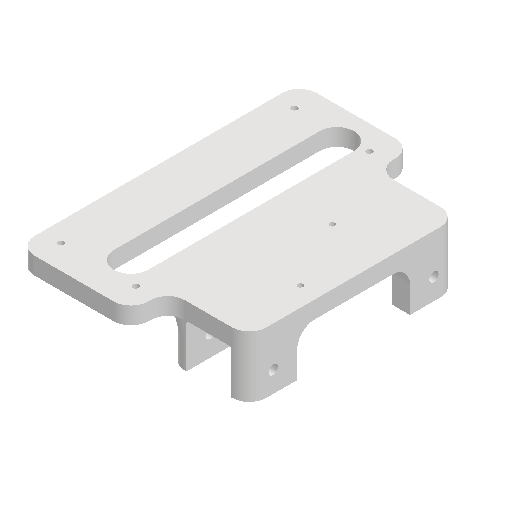
# Autodesk Inventor part: odriveAndBatteryMountV1
Saved by Autodesk Inventor 2025 (Build 290162000, 162)
## iProperties
Created: 2024-11-21
Part Number: odriveAndBatteryMountV1
Material: Generic
Document SubType Name: Modeling
Designer: derm
Density: 1 g/cm^3
Appearance: Default
Author: derm
Autodesk Inventor part; units mm, degrees
ref_plane "YZ Plane" through (0, 0, 0) normal (1, 0, 0) x (0, 1, 0)
ref_plane "XZ Plane" through (0, 0, 0) normal (0, 1, 0) x (-1, 0, 0)
ref_plane "XY Plane" through (0, 0, 0) normal (0, 0, 1) x (1, 0, 0)
sketch "Sketch1" plane through (0, 0, 0) normal (0, 1, 0) x (-1, 0, 0)
  line L0 (-21.75, 67.75) -> (21.75, 67.75) construction
  line L1 (21.75, 67.75) -> (21.75, -67.75) construction
  line L2 (21.75, -67.75) -> (-21.75, -67.75) construction
  line L3 (-21.75, -67.75) -> (-21.75, 67.75) construction
  line L4 (-21.75, 67.75) -> (21.75, -67.75) construction
  line L5 (21.75, 67.75) -> (-21.75, -67.75) construction
  line L6 (-32.9476, 81.798) -> (32.9476, 81.798)
  line L7 (32.9476, 81.798) -> (32.9476, -81.798)
  line L8 (32.9476, -81.798) -> (-32.9476, -81.798)
  line L9 (-32.9476, -81.798) -> (-32.9476, 81.798)
  line L10 (-32.9476, 81.798) -> (32.9476, -81.798) construction
  line L11 (32.9476, 81.798) -> (-32.9476, -81.798) construction
  circle A0 centre (21.75, 67.75) radius 1.75
  circle A1 centre (21.75, -67.75) radius 1.75
  circle A2 centre (-21.75, -67.75) radius 1.75
  circle A3 centre (-21.75, 67.75) radius 1.75
  line L12 (-31.798, -14.291) -> (-32.9476, -81.798)
  line L13 (-80.267, 60.5024) -> (-32.585, 60.5024)
  line L14 (-32.585, 60.5024) -> (-32.585, -60.5024)
  line L15 (-32.585, -60.5024) -> (-80.267, -60.5024)
  line L16 (-80.267, -60.5024) -> (-80.267, 60.5024)
  line L17 (-80.267, 60.5024) -> (-32.585, -60.5024) construction
  line L18 (-32.585, 60.5024) -> (-80.267, -60.5024) construction
  line L19 (-7.0609, 55.9115) -> (-7.0609, -63.5484) construction
  line L20 (-17.0051, 55.9115) -> (-17.0051, -63.5484)
  line L21 (2.8834, -63.5484) -> (2.8834, 55.9115)
  arc A4 (2.8834, 55.9115) -> (-17.0051, 55.9115) centre (-7.0609, 55.9115) ccw
  arc A5 (-17.0051, -63.5484) -> (2.8834, -63.5484) centre (-7.0609, -63.5484) ccw
  line L22 (32.9476, 81.798) -> (84.947, 81.798)
  line L23 (84.947, 81.798) -> (84.947, -81.798)
  line L24 (84.947, -81.798) -> (32.9476, -81.798)
  line L25 (32.9476, -81.798) -> (32.9476, 81.798)
  point P0 (0, 0)
  point P1 (-83.552, -67.75)
  point P2 (-56.426, 0)
  point P3 (-32.9476, -60.5024)
  point P4 (-32.9476, 60.5024)
  point P5 (-7.0609, -3.8185)
  dimension "d0" = 3.5
  dimension "d3" = 135.5
  dimension "d4" = 43.5
  constraints: 54 end point, 9 parallel, 7 midpoint, 6 centre point, 4 coincident, 4 horizontal, 4 perpendicular, 4 point on circle, 4 tangent, 3 equal radius, 2 point on line, 1 vertical, 1 other
  measures "d0" diameter of A3
  measures "d3" distance of L2.end L0.start
  measures "d4" distance of L0.start L0.end
extrude "Extrusion1" add sketch "Sketch1" against normal blind 10 contours L6 L7 L8 L12 L14 L13 L9 | L13 L14 L15 L9 | L9 L15 L16 L13
sketch "Sketch2" plane through (0, 0, 0) normal (0, 1, 0) x (1, 0, 0)
  circle A0 centre (69.0156, -19.6674) radius 1.6 projected
  circle A1 centre (47.6156, 20.3326) radius 1.6 projected
  point P0 (0, 0)
extrude "Extrusion2" cut sketch "Sketch2" against normal through all
sketch "Sketch3" plane through (0, -10, 0) normal (0, -1, 0) x (1, 0, 0)
  circle A0 centre (47.6156, -20.3326) radius 1.6 projected
  circle A1 centre (69.0156, 19.6674) radius 1.6 projected
  line L0 (32.585, -60.5024) -> (80.267, -60.5024) projected
  line L1 (80.267, -60.5024) -> (80.267, 60.5024) projected
  line L2 (80.267, 60.5024) -> (32.9476, 60.5024) projected
  line L3 (32.9476, 60.5024) -> (32.9476, 81.798) projected
  line L4 (32.9476, 81.798) -> (-32.9476, 81.798) projected
  line L5 (-32.9476, 81.798) -> (-32.9476, -81.798) projected
  line L6 (-32.9476, -81.798) -> (32.9476, -81.798) projected
  line L7 (32.9476, -81.798) -> (32.585, -60.5024) projected
  arc A2 (17.0051, 55.9115) -> (-2.8834, 55.9115) centre (7.0609, 55.9115) ccw projected
  line L8 (17.0051, 55.9115) -> (17.0051, -63.5484) projected
  arc A3 (-2.8834, -63.5484) -> (17.0051, -63.5484) centre (7.0609, -63.5484) ccw projected
  line L9 (-2.8834, -63.5484) -> (-2.8834, 55.9115) projected
  circle A4 centre (21.75, 67.75) radius 1.75 projected
  circle A5 centre (21.75, -67.75) radius 1.75 projected
  circle A6 centre (-21.75, -67.75) radius 1.75 projected
  circle A7 centre (-21.75, 67.75) radius 1.75 projected
  line L10 (69.6053, -60.5024) -> (43.8053, -60.5024)
  line L11 (43.8053, -60.5024) -> (43.8053, 60.5024)
  line L12 (43.8053, 60.5024) -> (69.6053, 60.5024)
  line L13 (69.6053, 60.5024) -> (69.6053, -60.5024)
  line L14 (69.6053, -60.5024) -> (43.8053, 60.5024) construction
  line L15 (43.8053, -60.5024) -> (69.6053, 60.5024) construction
  line L16 (80.5463, -32.7211) -> (32.8644, -32.7211)
  line L17 (32.8644, -32.7211) -> (32.8644, 32.7211)
  line L18 (32.8644, 32.7211) -> (80.5463, 32.7211)
  line L19 (80.5463, 32.7211) -> (80.5463, -32.7211)
  line L20 (80.5463, -32.7211) -> (32.8644, 32.7211) construction
  line L21 (32.8644, -32.7211) -> (80.5463, 32.7211) construction
  line L22 (32.8644, -32.7211) -> (32.6682, -32.7211)
  line L23 (32.585, -60.5024) -> (32.6682, -32.7211)
  line L24 (32.8644, 32.7211) -> (32.9476, 60.5024)
  point P0 (0, 0)
  point P1 (56.7053, 0)
  point P2 (80.267, -32.7211)
  point P3 (69.6053, -32.7211)
  point P4 (43.8053, -32.7211)
  point P5 (69.6053, 32.7211)
  point P6 (80.267, 32.7211)
  point P7 (43.8053, 32.7211)
  dimension "d7" = 25.8
  constraints: 30 end point, 4 midpoint, 4 parallel, 2 horizontal, 2 perpendicular, 2 point on line
  measures "d7" distance between parallel lines of L11 L13
extrude "Extrusion3" add sketch "Sketch3" along normal blind 25.4 contours L13 L2 L1 L18 | L16 L1 L0 L13 | L18 L24 L2 L11 | L11 L0 L23 L22 L16
fillet "Fillet1" radius 10 8 edges at (38.2368, -10, -32.7211) (38.3348, -10, 32.7211) (74.9362, -10, 32.7211) (74.9362, -10, -32.7211) (32.6682, -22.7, -32.7211) (32.6266, -10, -46.6118) (32.8644, -22.7, 32.7211) (32.906, -10, 46.6118)
fillet "Fillet2" radius 10 12 edges at (32.585, -5, -60.5024) (32.585, -27.7, -60.5024) (29.656, -12.9289, -60.5024) (32.9476, -5, -81.798) (-32.9476, -5, -81.798) (-32.9476, -5, 81.798) (32.9476, -5, 81.798) (32.9476, -5, 60.5024) (32.9476, -27.7, 60.5024) (30.0187, -12.9289, 60.5024) (80.267, -17.7, -60.5024) (80.267, -17.7, 60.5024)
fillet "Fillet3" radius 1 8 edges at (43.8053, -10, -27.7211) (43.8053, -10, -46.6118) (43.8053, -10, 27.7211) (43.8053, -10, 46.6118) (69.6053, -10, -27.7211) (69.6053, -10, -46.6118) (69.6053, -10, 46.6118) (69.6053, -10, 27.7211)
sketch "Sketch4" plane through (43.8053, -35.4, -32.7211) normal (1, 0, 0) x (0, 0, -1)
  line L0 (-93.2235, 24.4) -> (-59.8011, 24.4) projected
  line L1 (-93.2235, 24.4) -> (-93.2235, 0) projected
  line L2 (-65.4422, 0) -> (-93.2235, 0) projected
  line L3 (-65.4422, 15.4) -> (-65.4422, 0) projected
  arc A0 (-59.8011, 24.4) -> (-65.4422, 15.4) centre (-55.4422, 15.4) ccw projected
  line L4 (-5.6411, 24.4) -> (27.7813, 24.4) projected
  arc A1 (0, 15.4) -> (-5.6411, 24.4) centre (-10, 15.4) ccw projected
  line L5 (0, 15.4) -> (0, 0) projected
  line L6 (27.7813, 0) -> (0, 0) projected
  line L7 (27.7813, 24.4) -> (27.7813, 0) projected
  line L8 (-88.6326, 25.4) -> (30.8273, 25.4) projected
  circle A2 centre (13.8907, 12.2) radius 2.75
  circle A3 centre (-79.3329, 12.2) radius 2.75
  point P0 (-32.7211, 35.4)
  dimension "d13" = 5.5
  constraints: 2 centre point
  measures "d13" diameter of A2
extrude "Extrusion4" cut sketch "Sketch4" along normal through all both and the other way through all contours A2 | A3
body "Solid1"
